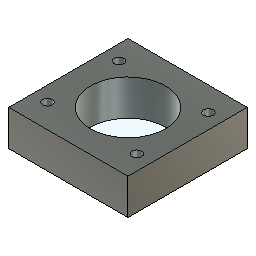
Motor Lifter (Autodesk Fusion 360 design; units mm, degrees)
Autodesk Fusion 360 part; units mm, degrees
sketch "Sketch1" plane through (0, 0, 0) normal (0, 0, 1) x (1, 0, 0)
  line L0 (-20, 20) -> (20, 20)
  line L1 (20, 20) -> (20, -20)
  line L2 (20, -20) -> (-20, -20)
  line L3 (-20, -20) -> (-20, 20)
  line L4 (0, 0) -> (15, 0)
  line L5 (0, 0) -> (0, -12)
  line L6 (0, -12) -> (15, -12)
  line L7 (15, -12) -> (-15, -12)
  line L8 (-15, -12) -> (-15, 12)
  line L9 (-15, 12) -> (15, 12)
  line L10 (15, 12) -> (15, -12)
  circle A0 centre (-15, 12) radius 1.5
  circle A1 centre (15, 12) radius 1.5
  circle A2 centre (15, -12) radius 1.5
  circle A3 centre (-15, -12) radius 1.5
  dimension "d1" = 12
  dimension "d2" = 30
  dimension "d3" = 24
  dimension "d4" = 3
  dimension "d5" = 3
  dimension "d6" = 3
  dimension "d7" = 3
  constraint horizontal L0
  constraint vertical L1
  constraint horizontal L2
  constraint vertical L3
  constraint coincident L4.start L5.start
  constraint perpendicular L3 L4
  constraint perpendicular L4 L5
  constraint perpendicular L5 L6
  constraint horizontal L7
  constraint vertical L8
  constraint horizontal L9
  constraint vertical L10
  constraint coincident L8.end L9.start
  constraint coincident L9.end L10.start
  constraint coincident L6.end L7.start
  constraint coincident L7.end L8.start
  measures "d1" distance of L4.start L5.end
  measures "d2" distance of L6.end L7.end
  measures "d3" distance of L6.end L9.end
  measures "d4" diameter of A0
  measures "d5" diameter of A1
  measures "d6" diameter of A2
  measures "d7" diameter of A3
extrude "Extrude1" add sketch "Sketch1" along normal blind 12 contours L0 L1 L2 L3 | L4 L5 L7 L8 L9 L10 A0 A1 A3 | L4 L5 L6 L7 L10 A2
sketch "Sketch2" plane through (0, 0, 12) normal (0, 0, 1) x (-1, 0, 0)
  circle A0 centre (-15, -12) radius 1.5
  circle A1 centre (15, 12) radius 1.5
  circle A2 centre (15, -12) radius 1.5
  circle A3 centre (-15, 12) radius 1.5
  line L0 (20, 20) -> (-20, 20)
  line L1 (-20, 20) -> (-20, -20)
  line L2 (-20, -20) -> (20, -20)
  line L3 (20, -20) -> (20, 20)
  circle A4 centre (0, 0) radius 12.5
  dimension "d10" = 25
  constraint coincident A4.centre origin
  measures "d10" diameter of A4
extrude "Extrude2" cut sketch "Sketch2" against normal blind 12 contours A4
sketch "Sketch3" plane through (0, 0, 12) normal (0, 0, 1) x (-1, 0, 0)
  circle A0 centre (0, 0) radius 12.5
  circle A1 centre (-15, -12) radius 1.5
  circle A2 centre (15, 12) radius 1.5
  circle A3 centre (15, -12) radius 1.5
  circle A4 centre (-15, 12) radius 1.5
  line L0 (20, 20) -> (-20, 20)
  line L1 (-20, 20) -> (-20, -20)
  line L2 (-20, -20) -> (20, -20)
  line L3 (20, -20) -> (20, 20)
  circle A5 centre (15, -12) radius 1.6
  circle A6 centre (-15, -12) radius 1.6
  circle A7 centre (-15, 12) radius 1.6
  circle A8 centre (15, 12) radius 1.6
  dimension "d13" = 3.2
  dimension "d14" = 3.2
  dimension "d15" = 3.2
  dimension "d16" = 3.2
  constraint concentric A3 A5
  constraint concentric A1 A6
  constraint concentric A4 A7
  constraint concentric A2 A8
  measures "d13" diameter of A5
  measures "d14" diameter of A6
  measures "d15" diameter of A7
  measures "d16" diameter of A8
extrude "Extrude3" cut sketch "Sketch3" against normal blind 12 contours A5 | A6 | A7 | A8
sketch "Sketch4" plane through (0, 0, 12) normal (0, 0, 1) x (-1, 0, 0)
  circle A0 centre (15, 12) radius 1.6
  circle A1 centre (-15, 12) radius 1.6
  circle A2 centre (15, -12) radius 1.6
  circle A3 centre (-15, -12) radius 1.6
  circle A4 centre (0, 0) radius 12.5
  line L0 (20, 20) -> (-20, 20)
  line L1 (-20, 20) -> (-20, -20)
  line L2 (-20, -20) -> (20, -20)
  line L3 (20, -20) -> (20, 20)
